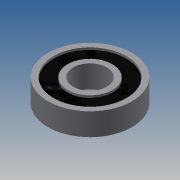
# Autodesk Inventor part: rodamiento
Saved by Autodesk Inventor 2017 (Build 210142000, 142)
## iProperties
Part Number: rodamiento
Material: Genérico
Document SubType Name: Modeling
Designer: FABLAB
Density: 1 g/cm^3
Appearance: Valor por defecto
Author: FABLAB
Autodesk Inventor part; units mm, degrees
ref_plane "YZ Plane" through (0, 0, 0) normal (1, 0, 0) x (0, 1, 0)
ref_plane "XZ Plane" through (0, 0, 0) normal (0, 1, 0) x (-1, 0, 0)
ref_plane "XY Plane" through (0, 0, 0) normal (0, 0, 1) x (1, 0, 0)
sketch "Boceto1" plane through (0, 0, 0) normal (1, 0, 0) x (0, 1, 0)
  line L0 (0, 30.1209) -> (0, -30.1209) construction
  line L1 (15, 4) -> (15, -4)
  line L2 (15, -4) -> (13, -4)
  line L3 (13, -4) -> (13, -3.2)
  line L4 (13, -3.2) -> (8, -3.2)
  line L5 (8, -3.2) -> (8, -4)
  line L6 (8, -4) -> (6, -4)
  line L7 (6, -4) -> (6, 4)
  line L8 (6, 4) -> (8, 4)
  line L9 (8, 4) -> (8, 3.2)
  line L10 (8, 3.2) -> (13, 3.2)
  line L11 (13, 3.2) -> (13, 4)
  line L12 (15, 4) -> (13, 4)
  circle A0 centre (10.5, 0) radius 2.2
  point P0 (0, 0)
  point P1 (0, 0)
  point P2 (6, 0)
  point P3 (10.5, -3.2)
  dimension "d0" = 1
  dimension "d1" = 0.3
  dimension "d2" = 30
  dimension "d3" = 8
  dimension "d4" = 0.8
  dimension "d5" = 2
  dimension "d6" = 12
  constraints: 26 end point, 7 perpendicular, 5 point on line, 3 equal length, 3 midpoint, 2 horizontal alignment, 2 vertical, 1 centre point, 1 coincident, 1 horizontal, 1 parallel, 1 vertical alignment
  measures "d0" distance edge to line of A0 L10
  measures "d1" distance edge to line of A0 L11
  measures "d2" diameter of L1 L0
  measures "d3" distance of L1.start L1.end
  measures "d4" distance of L10.end L11.end
  measures "d5" distance of L1.start L11.end
  measures "d6" diameter of L7 L0
revolve "Revolución1" add sketch "Boceto1" angle 360 about axis through (0, 0, 30.1209) along (0, 0, -1)
